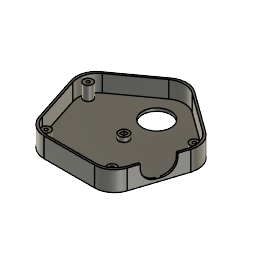
bottom_cover (Autodesk Fusion 360 design; units mm, degrees)
Autodesk Fusion 360 part; units mm, degrees
sketch "Sketch1" plane through (0, 0, 0) normal (0, 0, 1) x (1, 0, 0)
  line L0 (-62.3052, 20.2442) -> (-38.5068, -53)
  circle A0 centre (31.3849, 10.1976) radius 14.25 construction
  line L1 (38.5068, -53) -> (62.3052, 20.2442)
  line L2 (62.3052, 20.2442) -> (0, 65.5116)
  line L3 (-38.5068, -53) -> (38.5068, -53)
  circle A1 centre (0, 0) radius 50 construction
  circle A2 centre (19.3969, -26.6976) radius 14.25 construction
  circle A3 centre (-31.3849, 10.1976) radius 14.25 construction
  circle A4 centre (50.406, -16.3779) radius 15 construction
  circle A5 centre (0, 33) radius 14.25
  line L4 (0, 65.5116) -> (-62.3052, 20.2442)
  circle A6 centre (-19.3969, -26.6976) radius 14.25 construction
  line L5 (-39.9598, -55) -> (39.9598, -55)
  line L6 (39.9598, -55) -> (64.6564, 21.0081)
  line L7 (64.6564, 21.0081) -> (0, 67.9837)
  line L8 (0, 67.9837) -> (-64.6564, 21.0081)
  line L9 (-64.6564, 21.0081) -> (-39.9598, -55)
  line L10 (-37.0537, -51) -> (37.0537, -51) construction
  line L11 (37.0537, -51) -> (59.9541, 19.4803) construction
  line L12 (59.9541, 19.4803) -> (0, 63.0395) construction
  line L13 (0, 63.0395) -> (-59.9541, 19.4803) construction
  line L14 (-59.9541, 19.4803) -> (-37.0537, -51) construction
  line L15 (0, 0) -> (-59.9541, 19.4803) construction
  circle A7 centre (-53.2925, 17.3158) radius 1.6
  line L16 (-49.9041, 18.036) -> (-52.2221, 20.6103)
  line L17 (-52.2221, 20.6103) -> (-55.6105, 19.8901)
  line L18 (-55.6105, 19.8901) -> (-56.6809, 16.5956)
  line L19 (-56.6809, 16.5956) -> (-54.363, 14.0212)
  line L20 (-54.363, 14.0212) -> (-50.9746, 14.7415)
  line L21 (-50.9746, 14.7415) -> (-49.9041, 18.036)
  circle A8 centre (-53.2925, 17.3158) radius 4.5
  circle A9 centre (0, 0) radius 5
  line L22 (2.1, -2.1) -> (-2.1, -2.1)
  line L23 (-2.1, -2.1) -> (-2.1, 2.1)
  line L24 (-2.1, 2.1) -> (2.1, 2.1)
  line L25 (2.1, 2.1) -> (2.1, -2.1)
  line L26 (2.1, -2.1) -> (-2.1, 2.1) construction
  line L27 (-2.1, -2.1) -> (2.1, 2.1) construction
  point P0 (-53.2925, 17.3158)
  dimension "d2" = 360
  dimension "d4" = 53
  dimension "d5" = 100
  dimension "d6" = 28.5
  dimension "d7" = 33
  dimension "d8" = 30
  dimension "d9" = 2
  dimension "d10" = -2
  dimension "d37" = 3.2
  dimension "d38" = 63.0395
  dimension "d39" = 7.0044
  dimension "d40" = 3
  dimension "d41" = 9
  dimension "d51" = 10
  dimension "d52" = 4.2
  dimension "d53" = 4.2
  constraint coincident A1.centre L15.start
  constraint vertical A5.centre A1.centre
  constraint midpoint A4.centre L1
  constraint coincident L15 P0
  constraint coincident P0 A7.centre
  constraint horizontal L22
  constraint perpendicular L22 L23
  constraint parallel L22 L24
  constraint parallel L23 L25
  constraint coincident L26 A1.centre
  constraint coincident L27 A1.centre
  measures "d4" distance of A1.centre L3
  measures "d5" diameter of A1
  measures "d6" diameter of A5
  measures "d7" distance of A5.centre A1.centre
  measures "d8" diameter of A4
  measures "d37" diameter of A7
  measures "d38" distance of A1.centre L13.end
  measures "d39" distance of L13.end P0
  measures "d40" distance of P0 L21
  measures "d41" diameter of A8
  measures "d51" diameter of A9
  measures "d52" distance of L23.end L24.end
  measures "d53" distance of L22.end L23.end
extrude "Extrude1" add sketch "Sketch1" along normal blind 3 contours L0 L1 L2 L3 L4 | A7 | L16 L17 L18 L19 L20 L21 | A8 | A9 | L22 L23 L24 L25
extrude "Extrude2" add sketch "Sketch1" along normal blind 20 contours L5 L6 L7 L8 L9
sketch "Sketch3" plane through (52.3081, -16.9959, 0) normal (0.951057, -0.309017, 0) x (0.309017, 0.951057, 0)
  line L0 (-39.9598, 0) -> (39.9598, 0)
  line L1 (39.9598, 0) -> (39.9598, 20)
  line L2 (39.9598, 20) -> (-39.9598, 20)
  line L3 (-39.9598, 20) -> (-39.9598, 0)
  line L4 (-15, 20) -> (15, 20)
  line L5 (15, 20) -> (15, 3)
  line L6 (15, 3) -> (-15, 3)
  line L7 (-15, 3) -> (-15, 20)
  dimension "d22" = 30
  dimension "d23" = 17
  dimension "d24" = 15
  constraint horizontal L4
  constraint vertical L5
  constraint horizontal L6
  constraint vertical L7
  constraint coincident L2 L4.start
  measures "d22" distance of L4.start L4.end
  measures "d23" distance of L4.start L6.end
  measures "d24" horizontal distance of origin L6.end
extrude "Extrude4" cut sketch "Sketch3" against normal blind 2 contours L2 L4 L5 L6 L7
fillet "Fillet3" radius 13 2 edges at (46.7218, -30.9528, 3) (55.9923, -2.4211, 3)
fillet "Fillet3" radius 20 5 edges at (-62.3052, 20.2442, 11.5) (-38.5068, -53, 11.5) (38.5068, -53, 11.5) (62.3052, 20.2442, 11.5) (0, 65.5116, 11.5)
fillet "Fillet3" radius 20 5 edges at (-39.9598, -55, 10) (39.9598, -55, 10) (64.6564, 21.0081, 10) (0, 67.9837, 10) (-64.6564, 21.0081, 10)
extrude "Extrude5" add sketch "Sketch1" along normal blind 17 contours L16 L17 L18 L19 L20 L21 | A8
extrude "Extrude6" cut sketch "Sketch1" along normal blind 2 contours L16 L17 L18 L19 L20 L21
extrude "Extrude7" cut sketch "Sketch1" along normal blind 3 contours A7
pattern_circular "C-Pattern1" count 4 over 216.5 about axis through (0, 0, 1.75) along (0, 0, 1) of "Extrude5", "Extrude6", "Extrude7"
extrude "Extrude8" add sketch "Sketch1" along normal blind 4.5 from surface at 3 contours A9 | L22 L23 L24 L25
extrude "Extrude9" cut sketch "Sketch1" against normal blind 3.5 from surface at 7.5 contours L22 L23 L24 L25
equation "d39 = d38 / 9"
